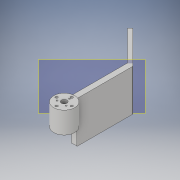
# Autodesk Inventor part: палец
Saved by Autodesk Inventor 2019 (Build 230136000, 136)
## iProperties
Created: 2019-08-15
Part Number: палец
Material: Типовые
Document SubType Name: Modeling
Designer: Петров Иван
Density: 1 g/cm^3
Appearance: По умолчанию
Author: Петров Иван
Autodesk Inventor part; units mm, degrees
ref_plane "YZ Plane" through (0, 0, 0) normal (1, 0, 0) x (0, 1, 0)
ref_plane "XZ Plane" through (0, 0, 0) normal (0, 1, 0) x (-1, 0, 0)
ref_plane "XY Plane" through (0, 0, 0) normal (0, 0, 1) x (1, 0, 0)
sketch "Эскиз1" plane through (0, 0, 0) normal (0, 1, 0) x (-1, 0, 0)
  arc A0 (-0.25, 9.2247) -> (0.25, 9.2247) centre (0, 8) ccw
  line L0 (-0.25, 10.9972) -> (-0.25, 9.2247)
  arc A1 (-0.25, 10.9972) -> (-1.1469, -10.94) centre (0, 0) ccw
  line L1 (-1.1469, -10.6297) -> (-1.1469, -10.94)
  line L2 (-0.8473, -10.6297) -> (-1.1469, -10.6297)
  line L3 (-0.8473, -10.9673) -> (-0.8473, -10.6297)
  arc A2 (-0.8473, -10.9673) -> (0.8535, -10.9668) centre (0, 0) ccw
  line L4 (0.8535, -10.6297) -> (0.8535, -10.9668)
  line L5 (1.1541, -10.6297) -> (0.8535, -10.6297)
  line L6 (1.1541, -10.9393) -> (1.1541, -10.6297)
  arc A3 (1.1541, -10.9393) -> (0.25, 10.9972) centre (0, 0) ccw
  line L7 (0.25, 9.2247) -> (0.25, 10.9972)
  circle A4 centre (8, 0) radius 1.25
  circle A5 centre (0, -8) radius 1.25
  circle A6 centre (-8, 0) radius 1.25
  circle A7 centre (0, -5.5) radius 0.75
  circle A8 centre (4.7631, 2.75) radius 0.75
  circle A9 centre (-4.7631, 2.75) radius 0.75
  circle A10 centre (0, 0) radius 2.9
  arc A11 (0.25, 9.2247) -> (-0.25, 9.2247) centre (0, 8) ccw
  circle A12 centre (0, 0) radius 11
  constraints: 16 end point, 13 centre point, 10 point on circle, 1 coincident, 1 concentric
extrude "Выдавливание1" add sketch "Эскиз1" along normal blind 22.76 contours A0 L7 A3 L6 L5 L4 A2 L3 L2 L1 A1 L0 | L0 A12 L7 A11 | L1 L2 L3 A12 | A12 L4 L5 L6
sketch "Эскиз2" plane through (0, 22.76, 0) normal (0, 1, 0) x (1, 0, 0)
  circle A0 centre (0, 0) radius 2.9 projected
  line L0 (-2.9, 0) -> (2.9, 0)
  line L1 (2.9, 0) -> (2.9, 19.5825)
  line L2 (2.9, 19.5825) -> (-2.9, 19.5825)
  line L3 (-2.9, 19.5825) -> (-2.9, 0)
  circle A1 centre (0, 0) radius 11 projected
  arc A2 (2.9, 10.6108) -> (-2.9, 10.6108) centre (0, 0) ccw
  constraints: 8 end point, 4 point on circle, 2 parallel, 2 point on line, 1 centre point, 1 horizontal, 1 horizontal alignment, 1 perpendicular, 1 other
extrude "Выдавливание2" add sketch "Эскиз2" against normal blind 22.76 contours A1 L3 L2 L1
sketch "Эскиз3" plane through (0, 22.76, 0) normal (0, 1, 0) x (1, 0, 0)
  line L0 (2.9, 19.5825) -> (2.9, 10.6108) projected
  arc A0 (2.9, 10.6108) -> (-2.9, 10.6108) centre (0, 0) ccw
  line L1 (-2.9, 19.5825) -> (-2.9, 10.6108) projected
  line L2 (-2.9, 10.6108) -> (2.9, 10.6108)
  line L3 (2.9, 10.6108) -> (2.9, 19.5825)
  line L4 (2.9, 19.5825) -> (-2.9, 19.5825)
  line L5 (-2.9, 19.5825) -> (-2.9, 10.6108)
  point P0 (0, 0)
  constraints: 8 end point, 2 parallel, 2 point on circle, 1 centre point, 1 horizontal, 1 perpendicular
extrude "Выдавливание3" cut sketch "Эскиз3" against normal blind 1 contours L0 A0 L1 L4
sketch "Эскиз4" plane through (0, 0, 0) normal (0, -1, 0) x (1, 0, 0)
  arc A0 (-2.9, -10.6108) -> (2.9, -10.6108) centre (0, 0) ccw projected
  arc A1 (-2.9, -10.6108) -> (2.9, -10.6108) centre (0, 0) ccw
  line L0 (-2.9, -10.6108) -> (-2.9, -19.5825) projected
  line L1 (2.9, -10.6108) -> (-2.9, -10.6108)
  line L2 (-2.9, -10.6108) -> (-2.9, -19.5825)
  line L3 (-2.9, -19.5825) -> (2.9, -19.5825)
  line L4 (2.9, -19.5825) -> (2.9, -10.6108)
  point P0 (0, 0)
  constraints: 8 end point, 2 parallel, 2 point on circle, 1 centre point, 1 horizontal, 1 perpendicular
extrude "Выдавливание4" add sketch "Эскиз4" along normal blind 22 contours A0 L4 L3 L0
move faces "Перенос1" translate (0, 0, -50) faces at (-0.9667, 7.1733, -19.5825)
ref_plane "РабПлоскость1" through (-2.9, -22, -69.5825) normal (-0.7071068, 0, -0.7071068) x (0, -1, 0)
sketch "Эскиз5" plane through (-2.9, -22, -69.5825) normal (-0.7071068, 0, -0.7071068) x (0, -1, 0)
  line L0 (-43.76, 0) -> (0, 0) projected
  line L1 (-43.76, -4.1012) -> (-43.76, 37.598) projected
  line L2 (0, 0) -> (-43.76, 0)
  line L3 (-43.76, 0) -> (-43.76, -4.1012)
  line L4 (-43.76, -4.1012) -> (0, -4.1012)
  line L5 (0, -4.1012) -> (0, 0)
  point P0 (-22, 47.1516)
  constraints: 8 end point, 2 parallel, 1 horizontal, 1 perpendicular
extrude "Выдавливание5" add sketch "Эскиз5" along normal blind 45 and the other way blind 4.25
